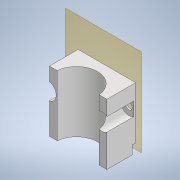
# Autodesk Inventor part: MotorBracket
Saved by Autodesk Inventor 2020.2 (Build 242310000, 310)
## iProperties
Created: 2020-04-18
Part Number: MotorBracket
Material: Generic
Document SubType Name: Modeling
Designer: Josiah
Density: 1 g/cm^3
Appearance: Default
Author: Josiah
Autodesk Inventor part; units mm, degrees
ref_plane "YZ Plane" through (0, 0, 0) normal (1, 0, 0) x (0, 1, 0)
ref_plane "XZ Plane" through (0, 0, 0) normal (0, 1, 0) x (-1, 0, 0)
ref_plane "XY Plane" through (0, 0, 0) normal (0, 0, 1) x (1, 0, 0)
sketch "Sketch1" plane through (0, 0, 0) normal (0, 0, 1) x (1, 0, 0)
  line L0 (10, -15) -> (-10, -15) projected
  line L1 (10, 15) -> (10, -15) projected
  line L2 (-10, 15) -> (10, 15) projected
  line L3 (-10, -15) -> (-10, 15) projected
  line L4 (9.6, -14.6) -> (-9.6, -14.6)
  line L5 (-9.6, -14.6) -> (-9.6, 14.6)
  line L6 (-9.6, 14.6) -> (9.6, 14.6)
  line L7 (9.6, 14.6) -> (9.6, -14.6)
  point P0 (0, 0)
  dimension "d0" = 0.4
  constraints: 8 end point, 3 other
  measures "d0" distance between parallel lines of L1 L7
ref_plane "Work Plane1" through (-20.5, -15, 1) normal (0, 0, 1) x (1, 0, 0)
extrude "Extrusion1" add sketch "Sketch1" along normal up to surface (1 mm away) contours L4 L5 L6 L7
sketch "Sketch2" plane through (-9.6, -14.6, 1) normal (0, 0, 1) x (1, 0, 0)
  circle A0 centre (-6.4, 18.6) radius 2 projected
  circle A1 centre (25.6, 18.6) radius 2 projected
  line L0 (0, 0) -> (0, 29.2) projected
  line L1 (19.2, 0) -> (0, 0) projected
  line L2 (19.2, 29.2) -> (19.2, 0) projected
  line L3 (0, 29.2) -> (19.2, 29.2) projected
  line L4 (-0.4, -4.9) -> (-0.4, 26.1) construction
  line L5 (23.6, -4.9) -> (23.6, 26.1) construction
  line L6 (28.6, 31.5) -> (-5.4, 31.5)
  line L7 (-5.4, 31.5) -> (-5.4, -4.5)
  line L8 (-5.4, -4.5) -> (28.6, -4.5)
  line L9 (28.6, -4.5) -> (28.6, 31.5)
  circle A2 centre (25.6, 18.6) radius 5
  circle A3 centre (-6.4, 18.6) radius 5
  point P0 (-5.4, 23.499)
  point P1 (-5.4, 13.701)
  point P2 (28.6, 14.6)
  point P3 (28.6, 22.6)
  dimension "d12" = 34
  dimension "d13" = 4.5
  dimension "d14" = 24
  dimension "d15" = 5
  dimension "d16" = 36
  dimension "d17" = 3
  dimension "d18" = 3
  constraints: 12 end point, 2 centre point, 2 parallel, 2 vertical, 1 horizontal, 1 perpendicular, 4 other
  measures "d12" distance of L6.start L6.end
  measures "d13" distance between parallel lines of L8 L1
  measures "d14" distance between parallel lines of L4 L5
  measures "d15" distance between parallel lines of L9 L5
  measures "d16" distance of L8.end L6.start
  measures "d17" radial gap between concentric circles of A1 A2
  measures "d18" radial gap between concentric circles of A0 A3
extrude "Extrusion2" add sketch "Sketch2" along normal blind 17 contours L7 L6 L9 A2 L8 A3 | L0 L3 L2 L1
sketch "Sketch4" plane through (-15, 16.9, 1) normal (0, 1, 0) x (1, 0, 0)
  circle A0 centre (17, -18) radius 12 projected
  circle A1 centre (17, -18) radius 12.4
  point P0 (15, 1)
  dimension "d19" = 0.4
  constraints: 1 centre point
  measures "d19" radial gap between concentric circles of A0 A1
extrude "Extrusion3" cut sketch "Sketch4" against normal up to surface (36 mm away) contours A0 | A1
ref_plane "Work Plane2" through (0, -91, 1) normal (0, 0, 1) x (1, 0, 0)
ref_plane "Work Plane3" through (0, -91, 1) normal (0, 0, 1) x (1, 0, 0)
sketch "Sketch5" plane through (0, -91, 1) normal (0, 0, 1) x (1, 0, 0)
  circle A0 centre (-16, 95) radius 2 projected
  circle A1 centre (16, 95) radius 2 projected
  line L0 (19, 99) -> (19, 107.9) projected
  line L1 (19, 102) -> (-19.6499, 102)
  line L2 (-19.6499, 102) -> (-19.6499, 88)
  line L3 (-19.6499, 88) -> (19, 88)
  line L4 (19, 88) -> (19, 102)
  point P0 (0, 91)
  dimension "d22" = 14
  dimension "d23" = 7
  dimension "d24" = 3.6498
  constraints: 8 end point, 2 parallel, 1 horizontal, 1 perpendicular, 1 point on line
  measures "d22" distance between parallel lines of L3 L1
  measures "d23" distance from line of L3 A0.centre
  measures "d24" distance from line of L2 A0.centre
extrude "Extrusion4" add sketch "Sketch5" along normal blind 1
sketch "Sketch6" plane through (-9.6, -14.6, 1) normal (0, 0, -1) x (-1, 0, 0)
  line L0 (-30.1, -0.4) -> (10.9, -0.4)
  line L1 (-28.6, -4.5) -> (-28.6, 31.5) projected
  line L2 (5.4, 11.6) -> (5.4, -4.5) projected
  line L3 (-28.6, 0.521) -> (5.4, 0.521)
  line L4 (5.4, 0.521) -> (5.4, -4.5)
  line L5 (5.4, -4.5) -> (-28.6, -4.5)
  line L6 (-28.6, -4.5) -> (-28.6, 0.521)
  point P0 (-9.6, 14.6)
  point P1 (5.4, 0.521)
  constraints: 10 end point, 2 horizontal, 2 parallel, 1 perpendicular, 1 point on line, 2 other
extrude "Extrusion5" cut sketch "Sketch6" against normal mid plane 4
equation "\"d15\" = -0.5 * d14 + 0.5 * d12"
equation "\"d23\" = 0.5 * d22"
body "Solid1"
